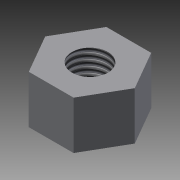
# Autodesk Inventor part: PulleyNut
Saved by Autodesk Inventor 2015 (Build 190159000, 159)
## iProperties
Created: 2017-01-05
Part Number: PulleyNut
Material: Generic
Document SubType Name: Modeling
Designer: Ernest
Density: 1 g/cm^3
Appearance: Default
Author: Ernest
Autodesk Inventor part; units mm, degrees
ref_plane "YZ Plane" through (0, 0, 0) normal (1, 0, 0) x (0, 1, 0)
ref_plane "XZ Plane" through (0, 0, 0) normal (0, 1, 0) x (-1, 0, 0)
ref_plane "XY Plane" through (0, 0, 0) normal (0, 0, 1) x (1, 0, 0)
sketch "Sketch1" plane through (0, 0, 0) normal (0, 0, 1) x (1, 0, 0)
  circle A0 centre (0, 0) radius 1.5
  line L0 (3.737, 0) -> (1.8685, -3.2364)
  line L1 (1.8685, -3.2364) -> (-1.8685, -3.2364)
  line L2 (-1.8685, -3.2364) -> (-3.737, 0)
  line L3 (-3.737, 0) -> (-1.8685, 3.2364)
  line L4 (-1.8685, 3.2364) -> (1.8685, 3.2364)
  line L5 (1.8685, 3.2364) -> (3.737, 0)
  dimension "d0" = 3
  constraints: 12 end point, 2 coincident, 1 centre point, 13 other
  measures "d0" diameter of A0
extrude "Extrusion1" add sketch "Sketch1" along normal blind 4
thread "Thread1" size "M3x0.5" class "6H" standard "ANSI Metric M Profile" full length
body "Solid1"
